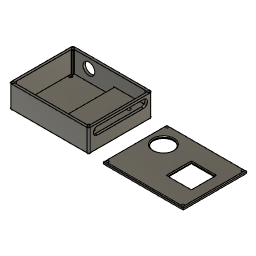
Caixa_pi_Pico (Autodesk Fusion 360 design; units mm, degrees)
Autodesk Fusion 360 part; units mm, degrees
sketch "Esboço1" plane through (0, 0, 0) normal (0, 0, 1) x (1, 0, 0)
  line L0 (0, 0) -> (0, 81)
  line L1 (0, 0) -> (101, 0)
  line L2 (0, 81) -> (101, 81)
  line L3 (101, 81) -> (101, 0)
  dimension "d1" = 81
  dimension "d2" = 101
  constraint coincident L0.start L1.start
  constraint vertical L0
  constraint perpendicular L0 L1
  constraint perpendicular L0 L2
  constraint perpendicular L1 L3
  measures "d1" distance of L0.start L0.end
  measures "d2" distance of L0.start L1.end
extrude "Extrusão2" add sketch "Esboço1" along normal blind 30 makes body 1
sketch "Esboço3" plane through (0, 0, 30) normal (0, 0, 1) x (-1, 0, 0)
  line L0 (0, 0) -> (-101, 0)
  line L1 (-101, 0) -> (-101, -81)
  line L2 (-101, -81) -> (0, -81)
  line L3 (0, -81) -> (0, 0)
  line L4 (-3, -2.9644) -> (-2.913, -77.9646)
  line L5 (-2.913, -77.9646) -> (-97.9408, -78.0749)
  line L6 (-97.9408, -78.0749) -> (-98.0278, -3.0746)
  line L7 (-98.0278, -3.0746) -> (-3, -2.9644)
  constraint perpendicular L4 L5
  constraint perpendicular L5 L6
  constraint perpendicular L6 L7
extrude "Extrusão3" cut sketch "Esboço3" against normal blind 27 contours L4 L5 L6 L7 bodies 1
hole "Furo1" at (23.413, 77.9884, 18) direction (-0.00116, 0.999999, 0) diameter 15 depth 10 tip angle 180 bodies 1
sketch "Esboço4" plane through (0, 0, 3) normal (0, 0, 1) x (-1, 0, 0)
  line L0 (-98.0278, -3.0746) -> (-97.9408, -78.0749)
  line L1 (-97.9408, -78.0749) -> (-2.913, -77.9646)
  line L2 (-2.913, -77.9646) -> (-3, -2.9644)
  line L3 (-3, -2.9644) -> (-98.0278, -3.0746)
  line L4 (-54.1357, -3.0237) -> (-54.0487, -78.024)
  constraint coincident L1 L4.end
  constraint perpendicular L1 L4
  constraint coincident L3 L4.start
extrude "Extrusão4" add sketch "Esboço4" along normal blind 11 contours L0 L1 L3 L4 bodies 1
sketch "Esboço5" plane through (98.0313, 0.1137, 0) normal (-0.999999, -0.00116, 0) x (0.00116, -0.999999, 0)
  line L0 (-77.9612, 14) -> (-2.9609, 14)
  line L1 (-2.9609, 14) -> (-2.9609, 30)
  line L2 (-2.9609, 30) -> (-77.9612, 30)
  line L3 (-77.9612, 30) -> (-77.9612, 14)
  line L4 (-5.9609, 27) -> (-74.9612, 27)
  line L5 (-74.9612, 27) -> (-74.9612, 17)
  line L6 (-74.9612, 17) -> (-5.9609, 17)
  line L7 (-5.9609, 17) -> (-5.9609, 27)
  constraint perpendicular L5 L6
  constraint perpendicular L4 L7
extrude "Extrusão5" cut sketch "Esboço5" against normal blind 110 contours L4 L5 L6 L7 bodies 1
fillet "Arredondamento1" radius 5 4 edges at (99.4722, 75.0767, 17) (99.4722, 75.0767, 27) (99.5122, 6.0764, 17) (99.5122, 6.0764, 27) on bodies 1
fillet "Arredondamento2" radius 2 9 edges at (101, 0, 15) (101, 40.5, 0) (50.5, 0, 0) (0, 0, 15) (101, 81, 15) (50.5, 81, 0) (0, 81, 15) (0, 40.5, 0) (54.0922, 40.5238, 14) on bodies 1
sketch "Esboço6" plane through (0, 0, 3) normal (0, 0, 1) x (-1, 0, 0)
  line L0 (-54.1357, -3.0237) -> (-54.0487, -78.024)
  line L1 (-54.0487, -78.024) -> (-2.913, -77.9646)
  line L2 (-2.913, -77.9646) -> (-3, -2.9644)
  line L3 (-3, -2.9644) -> (-54.1357, -3.0237)
  circle A0 centre (-51.308, -7.4889) radius 2
  circle A1 centre (-5.308, -7.4889) radius 2
  circle A2 centre (-5.308, -72.9889) radius 2
  circle A3 centre (-51.308, -72.9889) radius 2
  dimension "d38" = 65.5
  dimension "d39" = 46
  dimension "d40" = 4
  dimension "d41" = 4
  dimension "d42" = 4
  dimension "d43" = 4
  measures "d38" distance of A1.centre A2.centre
  measures "d39" distance of A0.centre A1.centre
  measures "d40" diameter of A0
  measures "d41" diameter of A1
  measures "d42" diameter of A2
  measures "d43" diameter of A3
extrude "Extrusão6" cut sketch "Esboço6" against normal blind 1.5 contours A0 | A1 | A2 | A3 bodies 1
sketch "Esboço7" plane through (0, 0, 14) normal (0, 0, 1) x (-1, 0, 0)
  line L0 (-56.0487, -78.0263) -> (-56.1357, -3.0261)
  line L1 (-56.1357, -3.0261) -> (-98.0278, -3.0746)
  line L2 (-98.0278, -3.0746) -> (-97.9408, -78.0749)
  line L3 (-97.9408, -78.0749) -> (-56.0487, -78.0263)
  circle A0 centre (-89.4363, -63.0726) radius 2
  circle A1 centre (-89.4363, -17.0726) radius 2
  dimension "d48" = 4
  dimension "d49" = 46
  dimension "d50" = 4
  measures "d48" diameter of A0
  measures "d49" distance of A0.centre A1.centre
  measures "d50" diameter of A1
extrude "Extrusão7" cut sketch "Esboço7" against normal blind 10 contours A0 | A1 bodies 1
sketch "Esboço8" plane through (0, 0, 30) normal (0, 0, 1) x (-1, 0, 0)
  line L0 (-2.913, -77.9646) -> (-97.9408, -78.0749)
  line L1 (-97.9408, -78.0749) -> (-98.0278, -3.0746)
  line L2 (-98.0278, -3.0746) -> (-3, -2.9644)
  line L3 (-3, -2.9644) -> (-2.913, -77.9646)
  arc A0 (-101, -79) -> (-99, -81) centre (-99, -79) ccw
  line L4 (-99, -81) -> (-2, -81)
  arc A1 (-2, -81) -> (0, -79) centre (-2, -79) ccw
  line L5 (0, -79) -> (0, -2)
  arc A2 (0, -2) -> (-2, 0) centre (-2, -2) ccw
  line L6 (-2, 0) -> (-99, 0)
  arc A3 (-99, 0) -> (-101, -2) centre (-99, -2) ccw
  line L7 (-101, -2) -> (-101, -79)
  line L8 (-95.9432, -78.0726) -> (-95.9432, -76.0633)
  line L9 (-95.9432, -76.0633) -> (-97.9432, -76.0633)
  line L10 (-96.0255, -3.0723) -> (-96.0255, -5.0723)
  line L11 (-96.0255, -5.0723) -> (-98.0255, -5.0723)
  constraint vertical L8
  constraint horizontal L9
  constraint coincident L0 L8.start
  constraint coincident L1 L9.end
  constraint coincident L8.end L9.start
  constraint vertical L10
  constraint perpendicular L10 L11
  constraint coincident L2 L10.start
  constraint coincident L1 L11.end
extrude "Extrusão8" add sketch "Esboço8" against normal blind 17 contours L0 L1 L8 L9 | L1 L2 L10 L11 bodies 1
fillet "Arredondamento3" radius 1 2 edges at (95.9432, 76.0633, 22) (96.0255, 5.0723, 22) on bodies 1
sketch "Esboço9" plane through (0, 0, 30) normal (0, 0, 1) x (-1, 0, 0)
  arc A0 (-101, -79) -> (-99, -81) centre (-99, -79) ccw
  line L0 (-99, -81) -> (-2, -81)
  arc A1 (-2, -81) -> (0, -79) centre (-2, -79) ccw
  line L1 (0, -79) -> (0, -2)
  arc A2 (0, -2) -> (-2, 0) centre (-2, -2) ccw
  line L2 (-2, 0) -> (-99, 0)
  arc A3 (-99, 0) -> (-101, -2) centre (-99, -2) ccw
  line L3 (-101, -2) -> (-101, -79)
  arc A4 (-97.0255, -5.0723) -> (-96.0255, -4.0723) centre (-97.0255, -4.0723) ccw
  line L4 (-96.0255, -4.0723) -> (-96.0255, -3.0723)
  line L5 (-96.0255, -3.0723) -> (-3, -2.9644)
  line L6 (-3, -2.9644) -> (-2.913, -77.9646)
  line L7 (-2.913, -77.9646) -> (-95.9432, -78.0726)
  line L8 (-95.9432, -78.0726) -> (-95.9432, -77.0633)
  arc A5 (-95.9432, -77.0633) -> (-96.9432, -76.0633) centre (-96.9432, -77.0633) ccw
  line L9 (-96.9432, -76.0633) -> (-97.9432, -76.0633)
  line L10 (-97.9432, -76.0633) -> (-98.0255, -5.0723)
  line L11 (-98.0255, -5.0723) -> (-97.0255, -5.0723)
  circle A6 centre (-98.5, -78.5) radius 1.5
  circle A7 centre (-98.5, -2.5) radius 1.5
  dimension "d63" = 3
  dimension "d64" = 3
  measures "d63" diameter of A6
  measures "d64" diameter of A7
extrude "Extrusão9" cut sketch "Esboço9" against normal blind 10 contours A6 | A7 bodies 1
sketch "Esboço10" plane through (0, 0, 3) normal (0, 0, 1) x (-1, 0, 0)
  circle A0 centre (-5.308, -7.4889) radius 2
  circle A1 centre (-5.308, -72.9889) radius 2
  circle A2 centre (-51.308, -7.4889) radius 2
  circle A3 centre (-51.308, -72.9889) radius 2
  line L0 (-54.1357, -3.0237) -> (-54.0487, -78.024)
  line L1 (-54.0487, -78.024) -> (-2.913, -77.9646)
  line L2 (-2.913, -77.9646) -> (-3, -2.9644)
  line L3 (-3, -2.9644) -> (-54.1357, -3.0237)
  line L4 (-2.9977, -4.9667) -> (-4.9977, -4.9667)
  line L5 (-4.9977, -4.9667) -> (-4.9977, -2.9667)
  line L6 (-2.9153, -75.967) -> (-4.9153, -75.967)
  line L7 (-4.9153, -75.967) -> (-4.9153, -77.967)
  dimension "d67" = 2
  dimension "d68" = 2
  dimension "d69" = 2
  dimension "d70" = 2
  constraint horizontal L4
  constraint perpendicular L4 L5
  constraint coincident L2 L4.start
  constraint coincident L3 L5.end
  constraint horizontal L6
  constraint perpendicular L6 L7
  constraint coincident L1 L7.end
  constraint coincident L2 L6.start
  measures "d67" distance of L4.start L4.end
  measures "d68" distance of L4.end L5.end
  measures "d69" distance of L6.start L6.end
  measures "d70" distance of L6.end L7.end
extrude "Extrusão10" add sketch "Esboço10" along normal blind 27 contours L2 L3 L4 L5 | L1 L2 L6 L7 bodies 1
fillet "Arredondamento4" radius 1 2 edges at (4.9977, 4.9667, 16.5) (4.9153, 75.967, 16.5) on bodies 1
sketch "Esboço11" plane through (0, 0, 30) normal (0, 0, 1) x (-1, 0, 0)
  circle A0 centre (-98.5, -78.5) radius 1.5
  circle A1 centre (-98.5, -2.5) radius 1.5
  arc A2 (-101, -79) -> (-99, -81) centre (-99, -79) ccw
  line L0 (-99, -81) -> (-2, -81)
  arc A3 (-2, -81) -> (0, -79) centre (-2, -79) ccw
  line L1 (0, -79) -> (0, -2)
  arc A4 (0, -2) -> (-2, 0) centre (-2, -2) ccw
  line L2 (-2, 0) -> (-99, 0)
  arc A5 (-99, 0) -> (-101, -2) centre (-99, -2) ccw
  line L3 (-101, -2) -> (-101, -79)
  arc A6 (-3.9153, -75.967) -> (-4.9153, -76.967) centre (-3.9153, -76.967) ccw
  line L4 (-4.9153, -76.967) -> (-4.9153, -77.967)
  line L5 (-4.9153, -77.967) -> (-95.9432, -78.0726)
  line L6 (-95.9432, -78.0726) -> (-95.9432, -77.0633)
  arc A7 (-95.9432, -77.0633) -> (-96.9432, -76.0633) centre (-96.9432, -77.0633) ccw
  line L7 (-96.9432, -76.0633) -> (-97.9432, -76.0633)
  line L8 (-97.9432, -76.0633) -> (-98.0255, -5.0723)
  line L9 (-98.0255, -5.0723) -> (-97.0255, -5.0723)
  arc A8 (-97.0255, -5.0723) -> (-96.0255, -4.0723) centre (-97.0255, -4.0723) ccw
  line L10 (-96.0255, -4.0723) -> (-96.0255, -3.0723)
  line L11 (-96.0255, -3.0723) -> (-4.9977, -2.9667)
  line L12 (-4.9977, -2.9667) -> (-4.9977, -3.9667)
  arc A9 (-4.9977, -3.9667) -> (-3.9977, -4.9667) centre (-3.9977, -3.9667) ccw
  line L13 (-3.9977, -4.9667) -> (-2.9977, -4.9667)
  line L14 (-2.9977, -4.9667) -> (-2.9153, -75.967)
  line L15 (-2.9153, -75.967) -> (-3.9153, -75.967)
  circle A10 centre (-2.5, -2.5) radius 1.5
  circle A11 centre (-2.5, -78.5) radius 1.5
  dimension "d75" = 3
  dimension "d76" = 3
  measures "d75" diameter of A10
  measures "d76" diameter of A11
extrude "Extrusão11" cut sketch "Esboço11" against normal blind 15 contours A10 | A11 bodies 1
sketch "Esboço12" plane through (0, 0, 0) normal (0, 0, 1) x (1, 0, 0)
  line L0 (221.3805, 84.0517) -> (119.7063, 84.0517)
  line L1 (221.3805, 84.0517) -> (221.3805, 3.0953)
  line L2 (221.3805, 3.0953) -> (119.7063, 3.0953)
  line L3 (119.7063, 84.0517) -> (119.7063, 3.0953)
  constraint horizontal L0
  constraint vertical L1
  constraint horizontal L2
  constraint vertical L3
  constraint coincident L0.end L3.start
  constraint coincident L0.start L1.start
  constraint coincident L1.end L2.start
  constraint coincident L2.end L3.end
extrude "Extrusão12" add sketch "Esboço12" along normal blind 3 separate body makes body 2
move_body "Mover1" bodies 2 to x (1, 0, 0) y (0, 1, 0) z (0, 0, 1) at (0, -3, 0)
sketch "Esboço13" plane through (0, 0, 3) normal (0, 0, 1) x (-1, 0, 0)
  line L0 (-221.3805, -81.0517) -> (-119.7063, -81.0517)
  line L1 (-119.7063, -81.0517) -> (-119.7063, -0.0953)
  line L2 (-119.7063, -0.0953) -> (-221.3805, -0.0953)
  line L3 (-221.3805, -0.0953) -> (-221.3805, -81.0517)
  circle A0 centre (-139.3754, -56.9697) radius 12.5
  line L4 (-206.3805, -55.5953) -> (-206.3805, -25.5953)
  line L5 (-206.3805, -25.5953) -> (-176.3805, -25.5953)
  line L6 (-176.3805, -25.5953) -> (-176.3805, -55.5953)
  line L7 (-176.3805, -55.5953) -> (-206.3805, -55.5953)
  circle A1 centre (-122.7349, -78.504) radius 1.5
  circle A2 centre (-218.7349, -78.504) radius 1.5
  circle A3 centre (-122.7349, -2.504) radius 1.5
  circle A4 centre (-218.7349, -2.504) radius 1.5
  constraint perpendicular L4 L5
  constraint perpendicular L4 L7
extrude "Extrusão13" cut sketch "Esboço13" against normal blind 20 contours A0 | L4 L5 L6 L7 | A1 | A2 | A3 | A4 bodies 2
fillet "Arredondamento5" radius 1 14 edges at (191.3805, 55.5953, 0) (191.3805, 55.5953, 3) (206.3805, 40.5953, 3) (206.3805, 40.5953, 0) (176.3805, 40.5953, 0) (176.3805, 40.5953, 3) (191.3805, 25.5953, 0) (191.3805, 25.5953, 3) (170.5434, 81.0517, 3) (221.3805, 40.5735, 3) (170.5434, 0.0953, 3) (119.7063, 40.5735, 3) (151.0295, 61.4899, 0) (151.0295, 52.4495, 3) on bodies 2
